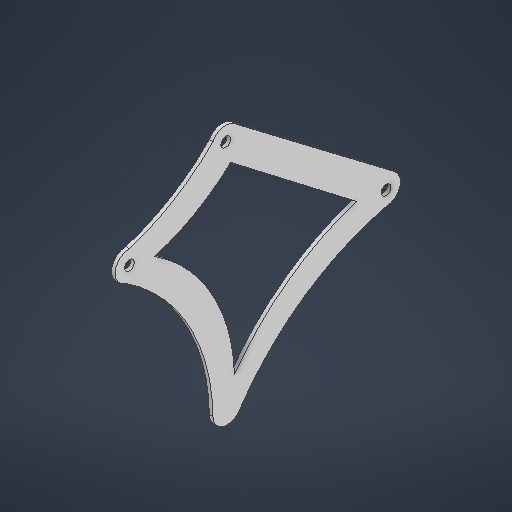
# Autodesk Inventor part: ringblockerv2
Saved by Autodesk Inventor 2025.2 (Build 292293000, 293)
## iProperties
Created: 2025-03-30
Part Number: ringblockerv2
Material: Generic
Document SubType Name: Modeling
Designer: roejo
Density: 1 g/cm^3
Appearance: Default
Author: roejo
Autodesk Inventor part; units mm, degrees
ref_plane "YZ Plane" through (0, 0, 0) normal (1, 0, 0) x (0, 1, 0)
ref_plane "XZ Plane" through (0, 0, 0) normal (0, 1, 0) x (-1, 0, 0)
ref_plane "XY Plane" through (0, 0, 0) normal (0, 0, 1) x (1, 0, 0)
sketch "Sketch1" plane through (0, 0, 0) normal (1, 0, 0) x (0, 1, 0)
  circle A0 centre (-50.3348, 10.4318) radius 6.35
  circle A1 centre (25.9635, 53.6322) radius 2.1844
  circle A2 centre (51.8593, 11.1419) radius 2.1844
  circle A3 centre (-1.8993, -59.6622) radius 2.1844
  arc A4 (-31.4874, -97.6281) -> (-30.8803, -97.2439) centre (-31.376, -97.1325) ccw
  line L0 (-31.4874, -97.6281) -> (-35.0063, -96.8369)
  arc A5 (-29.1899, -99.915) -> (-29.797, -100.2992) centre (-29.3014, -100.4107) ccw
  arc A6 (-31.4874, -97.6281) -> (-30.8803, -97.2439) centre (-31.376, -97.1325) ccw
  line L1 (-35.0063, -96.8369) -> (-31.4874, -97.6281)
  arc A7 (-37.6774, -98.5273) -> (-38.0616, -97.9203) centre (-38.1731, -98.4159) ccw
  line L2 (-38.0616, -97.9203) -> (-39.8211, -97.5246)
  arc A8 (-29.1899, -99.915) -> (-29.797, -100.2992) centre (-29.3014, -100.4107) ccw
  arc A9 (-37.6774, -98.5273) -> (-38.0616, -97.9203) centre (-38.1731, -98.4159) ccw
  line L3 (-39.8211, -97.5246) -> (-38.0616, -97.9203)
  line L4 (-39.8211, -97.5246) -> (-38.0616, -97.9203)
  arc A10 (-29.1899, -99.915) -> (-29.797, -100.2992) centre (-29.3014, -100.4107) ccw
  arc A11 (-37.6774, -98.5273) -> (-38.0616, -97.9203) centre (-38.1731, -98.4159) ccw
  arc A12 (-29.1899, -99.915) -> (-29.797, -100.2992) centre (-29.3014, -100.4107) ccw
  arc A13 (-31.4874, -97.6281) -> (-30.8803, -97.2439) centre (-31.376, -97.1325) ccw
  line L5 (-31.4874, -97.6281) -> (-35.0063, -96.8369)
  arc A14 (-37.6774, -98.5273) -> (-38.0616, -97.9203) centre (-38.1731, -98.4159) ccw
  line L6 (-38.0616, -97.9203) -> (-39.8211, -97.5246)
  arc A15 (-31.4874, -97.6281) -> (-30.8803, -97.2439) centre (-31.376, -97.1325) ccw
  line L7 (-35.0063, -96.8369) -> (-31.4874, -97.6281)
  circle A16 centre (25.9635, 53.6322) radius 6.35
  circle A17 centre (51.8593, 11.1419) radius 6.35
  circle A18 centre (-1.8993, -59.6622) radius 6.35
  arc A19 (-50.3348, 16.7818) -> (19.8389, 55.3092) centre (-51.5807, 102.222) ccw
  arc A20 (32.3135, 53.6322) -> (54.7772, 16.7818) centre (116.2711, 79.5401) ccw
  arc A21 (-8.2493, -59.6622) -> (-53.2527, 4.7919) centre (-114.0974, -85.6296) ccw
  line L8 (3.2531, -63.3736) -> (56.9166, 7.3019)
  arc A22 (-38.9414, 7.3019) -> (23.7791, 42.5126) centre (-41.3896, 85.1299) ccw
  arc A23 (23.7791, 42.5126) -> (42.9324, 8.9575) centre (103.5332, 65.7926) ccw
  line L9 (42.9324, 8.9575) -> (0.2851, -46.536)
  arc A24 (0.2851, -46.536) -> (-38.9414, 7.3019) centre (-100.9359, -79.0766) ccw
  point P0 (0, 0)
  dimension "d0" = 12.7
  dimension "d1" = 12.7
  dimension "d2" = 12.7
  dimension "d3" = 12.7
  constraints: 44 point on circle, 25 centre point, 20 end point, 3 coincident, 1 tangent
  measures "d0" diameter of A0
  measures "d1" diameter of A16
  measures "d2" diameter of A17
  measures "d3" diameter of A18
extrude "Extrusion1" add sketch "Sketch1" along normal blind 1.5875
body "Solid1"
